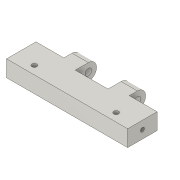
# Autodesk Inventor part: Lagerbock
Saved by Autodesk Inventor 2018.3 (Build 223284000, 284)
## iProperties
Created: 2019-11-28
Material: Stahl, unlegiert
Document SubType Name: Modeling
Designer: bauermeisterdi
Density: 7.85 g/cm^3
Appearance: Stahl
Description: Lagerbock
Werkstoff: S235JRC+C
Author: bauermeisterdi
Autodesk Inventor part; units mm, degrees
ref_plane "YZ Plane" through (0, 0, 0) normal (1, 0, 0) x (0, 1, 0)
ref_plane "XZ Plane" through (0, 0, 0) normal (0, 1, 0) x (-1, 0, 0)
ref_plane "XY Plane" through (0, 0, 0) normal (0, 0, 1) x (1, 0, 0)
sketch "Skizze_Grundkörper" plane through (0, 0, 0) normal (0, 0, 1) x (1, 0, 0)
  line L0 (-51.8, 0) -> (51.8, 0) projected
  line L1 (0, -19.6) -> (0, 19.6) projected
  line L2 (37, -14) -> (-37, -14)
  line L3 (-37, -14) -> (-37, 14)
  line L4 (-37, 14) -> (37, 14)
  line L5 (37, 14) -> (37, -14)
  line L6 (37, -14) -> (-37, 14) construction
  line L7 (-37, -14) -> (37, 14) construction
  point P0 (0, 0)
  dimension "Länge" = 74
  dimension "Höhe" = 28
  constraints: 12 end point, 2 midpoint, 2 parallel, 1 horizontal, 1 perpendicular
  measures "Länge" distance of L3.end L4.end
  measures "Höhe" distance of L4.end L2.start
extrude "Grundkörper" add sketch "Skizze_Grundkörper" along normal mid plane 10
sketch "Skizze_Ausnehmung_Mitte" plane through (0, 0, 5) normal (0, 0, 1) x (1, 0, 0)
  line L0 (-51.8, 0) -> (51.8, 0) projected
  line L1 (0, -19.6) -> (0, 19.6) projected
  line L2 (-37, -14) -> (37, -14) projected
  line L3 (37, -14) -> (37, 14) projected
  line L4 (37, 14) -> (-37, 14) projected
  line L5 (-37, 14) -> (-37, -14) projected
  line L6 (37, 14) -> (-37, 14) projected
  line L7 (10, 1) -> (-10, 1)
  line L8 (-10, 1) -> (-10, 14)
  line L9 (-10, 14) -> (10, 14)
  line L10 (10, 14) -> (10, 1)
  line L11 (10, 1) -> (-10, 14) construction
  line L12 (-10, 1) -> (10, 14) construction
  point P0 (0, 0)
  point P1 (0, 7.5)
  dimension "d4" = 20
  dimension "d5" = 13
  constraints: 12 end point, 2 midpoint, 2 parallel, 2 point on line, 1 horizontal, 1 perpendicular
  measures "d4" distance of L7.start L7.end
  measures "d5" distance of L9.end L7.start
extrude "Ausnehmung_Mitte" cut sketch "Skizze_Ausnehmung_Mitte" against normal through all contours L7 L8 L4 L1 | L1 L4 L10 L7
sketch "Skizze_Ausnehmung_Seite" plane through (0, 0, 5) normal (0, 0, 1) x (1, 0, 0)
  line L0 (-51.8, 0) -> (51.8, 0) projected
  line L1 (0, -19.6) -> (0, 19.6) projected
  line L2 (10, 14) -> (10, 1) projected
  line L3 (10, 1) -> (-10, 1) projected
  line L4 (-10, 1) -> (-10, 14) projected
  line L5 (-10, 14) -> (-37, 14) projected
  line L6 (-37, 14) -> (-37, -14) projected
  line L7 (-37, -14) -> (37, -14) projected
  line L8 (37, -14) -> (37, 14) projected
  line L9 (37, 14) -> (10, 14) projected
  line L10 (-37, 14) -> (-37, -14) projected
  line L11 (-37, 14) -> (-20, 14)
  line L12 (-20, 14) -> (-20, 4)
  line L13 (-20, 4) -> (-37, 4)
  line L14 (-37, 4) -> (-37, 14)
  line L15 (37, 14) -> (10, 14) projected
  line L16 (37, 14) -> (20, 14)
  line L17 (20, 14) -> (20, 4)
  line L18 (20, 4) -> (37, 4)
  line L19 (37, 4) -> (37, 14)
  point P0 (0, 0)
  dimension "d8" = 40
  dimension "d9" = 18
  constraints: 16 end point, 4 parallel, 2 horizontal, 2 perpendicular, 1 collinear, 1 other
  measures "d8" distance between parallel lines of L17 L12
  measures "d9" distance between parallel lines of L7 L18
extrude "Ausnehmung_Seite" cut sketch "Skizze_Ausnehmung_Seite" against normal through all contours L6 L5 L12 L13 | L18 L17 L9 L8
full round fillet "Rundung1" first side at (3.3333, -9, 5) centre faces at (-16.6667, 14, -1.6667) second side at (3.3333, -9, -5)
full round fillet "Rundung2" first side at (3.3333, -9, 5) centre faces at (13.3333, 14, -1.6667) second side at (3.3333, -9, -5)
hole "Bohrung_4_mm" at (-20, 9, 0) direction (1, 0, 0) diameter 4 end through all
sketch "Skizze_Bohrung_3_mm" plane through (0, 0, 5) normal (0, 0, 1) x (1, 0, 0)
  line L0 (-51.8, 0) -> (51.8, 0) projected
  line L1 (0, -19.6) -> (0, 19.6) projected
  line L2 (10, 9) -> (20, 9) projected
  line L3 (10, 9) -> (10, 1) projected
  line L4 (10, 1) -> (-10, 1) projected
  line L5 (-10, 1) -> (-10, 9) projected
  line L6 (-20, 9) -> (-10, 9) projected
  line L7 (-20, 9) -> (-20, 4) projected
  line L8 (-20, 4) -> (-37, 4) projected
  line L9 (-37, 4) -> (-37, -14) projected
  line L10 (-37, -14) -> (37, -14) projected
  line L11 (37, -14) -> (37, 4) projected
  line L12 (37, 4) -> (20, 4) projected
  line L13 (20, 4) -> (20, 9) projected
  point P0 (0, 0)
  point P1 (-25, -9)
  point P2 (25, -9)
  dimension "d21" = 50
  dimension "d22" = 5
  constraints: 1 symmetric about line
  measures "d21" distance of point (25, -9) point (-25, -9)
  measures "d22" distance from line of point (25, -9) L10
hole "Bohrung_3_mm" at (-25, -9, 5) at (25, -9, 5) direction (0, 0, -1) diameter 3 end through all
sketch "Skizze_M4" plane through (-37, -14, -5) normal (-1, 0, 0) x (0, 0, 1)
  line L0 (5, -5.6) -> (5, 33.6) projected
  line L1 (-2, 14) -> (12, 14) projected
  line L2 (10, 18) -> (0, 18) projected
  line L3 (0, 0) -> (0, 18) projected
  line L4 (10, 0) -> (0, 0) projected
  line L5 (10, 18) -> (10, 0) projected
  point P0 (5, 14)
  point P1 (5, 9)
  dimension "d30" = 9
  constraints: 1 point on line
  measures "d30" distance from line of point (5, 9) L4
hole "Bohrung_M4" at (-37, -5, 0) direction (1, 0, 0) diameter 2.459 depth 14 tip angle 118 thread size "M3x0.5" class "6H" standard "ISO Metric profile"
pattern_circular "Runde Anordnung_M4" count 2 over 360 about axis through (0, -10, 0) along (0, 1, 0) of "Bohrung_M4"
